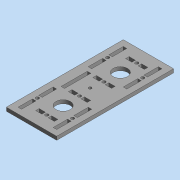
# Autodesk Inventor part: X-Anchor-Side
Saved by Autodesk Inventor 2016 SP1 (Build 200210100, 210)
## iProperties
Created: 2016-01-21
Part Number: X-Anchor-Side
Material: Generic
Document SubType Name: Modeling
Designer: Mohamed A.
Density: 1 g/cm^3
Appearance: Default
Author: Mohamed A.
Autodesk Inventor part; units mm, degrees
ref_plane "YZ Plane" through (0, 0, 0) normal (1, 0, 0) x (0, 1, 0)
ref_plane "XZ Plane" through (0, 0, 0) normal (0, 1, 0) x (-1, 0, 0)
ref_plane "XY Plane" through (0, 0, 0) normal (0, 0, 1) x (1, 0, 0)
sketch "Sketch1" plane through (0, 0, 0) normal (0, 0, 1) x (1, 0, 0)
  line L0 (21.5007, 49.9294) -> (-21.5007, 49.9294)
  line L1 (-21.5007, 49.9294) -> (-21.5007, -49.9294)
  line L2 (-21.5007, -49.9294) -> (21.5007, -49.9294)
  line L3 (21.5007, -49.9294) -> (21.5007, 49.9294)
  line L4 (-13.5007, 14.9765) -> (-16.5007, 14.9765)
  line L5 (-16.5007, 14.9765) -> (-16.5007, 27.3029)
  line L6 (-16.5007, 27.3029) -> (-13.5007, 27.3029)
  line L7 (-13.5007, 27.3029) -> (-13.5007, 14.9765)
  line L8 (-13.5007, -27.3029) -> (-16.5007, -27.3029)
  line L9 (-16.5007, -27.3029) -> (-16.5007, -14.9765)
  line L10 (-16.5007, -14.9765) -> (-13.5007, -14.9765)
  line L11 (-13.5007, -14.9765) -> (-13.5007, -27.3029)
  line L12 (-13.5007, -44.9294) -> (-16.5007, -44.9294)
  line L13 (-16.5007, -44.9294) -> (-16.5007, -32.6029)
  line L14 (-16.5007, -32.6029) -> (-13.5007, -32.6029)
  line L15 (-13.5007, -32.6029) -> (-13.5007, -44.9294)
  line L16 (-16.5007, 44.9294) -> (-13.5007, 44.9294)
  line L17 (-13.5007, 44.9294) -> (-13.5007, 32.6029)
  line L18 (-13.5007, 32.6029) -> (-16.5007, 32.6029)
  line L19 (-16.5007, 32.6029) -> (-16.5007, 44.9294)
  line L20 (-10.5007, -11.2324) -> (-13.5007, -11.2324)
  line L21 (-13.5007, -11.2324) -> (-13.5007, 11.2324)
  line L22 (-13.5007, 11.2324) -> (-10.5007, 11.2324)
  line L23 (-10.5007, 11.2324) -> (-10.5007, -11.2324)
  line L24 (16.5007, 14.9765) -> (13.5007, 14.9765)
  line L25 (13.5007, 14.9765) -> (13.5007, 27.3029)
  line L26 (13.5007, 27.3029) -> (16.5007, 27.3029)
  line L27 (16.5007, 27.3029) -> (16.5007, 14.9765)
  line L28 (16.5007, -27.3029) -> (13.5007, -27.3029)
  line L29 (13.5007, -27.3029) -> (13.5007, -14.9765)
  line L30 (13.5007, -14.9765) -> (16.5007, -14.9765)
  line L31 (16.5007, -14.9765) -> (16.5007, -27.3029)
  line L32 (16.5007, -44.9294) -> (13.5007, -44.9294)
  line L33 (13.5007, -44.9294) -> (13.5007, -32.6029)
  line L34 (13.5007, -32.6029) -> (16.5007, -32.6029)
  line L35 (16.5007, -32.6029) -> (16.5007, -44.9294)
  line L36 (13.5007, 44.9294) -> (16.5007, 44.9294)
  line L37 (16.5007, 44.9294) -> (16.5007, 32.6029)
  line L38 (16.5007, 32.6029) -> (13.5007, 32.6029)
  line L39 (13.5007, 32.6029) -> (13.5007, 44.9294)
  line L40 (4.1498, 36.9294) -> (4.1498, 39.9294)
  line L41 (4.1498, 39.9294) -> (9.5001, 39.9294)
  line L42 (9.5001, 39.9294) -> (9.5001, 36.9294)
  line L43 (9.5001, 36.9294) -> (4.1498, 36.9294)
  line L44 (-6.5006, 36.9294) -> (-6.5006, 39.9294)
  line L45 (-6.5006, 39.9294) -> (-1.1502, 39.9294)
  line L46 (-1.1502, 39.9294) -> (-1.1502, 36.9294)
  line L47 (-1.1502, 36.9294) -> (-6.5006, 36.9294)
  line L48 (-1.1502, 11.9294) -> (-1.1502, 8.9294)
  line L49 (-1.1502, 8.9294) -> (-6.5006, 8.9294)
  line L50 (-6.5006, 8.9294) -> (-6.5006, 11.9294)
  line L51 (-6.5006, 11.9294) -> (-1.1502, 11.9294)
  line L52 (9.5001, 11.9294) -> (9.5001, 8.9294)
  line L53 (9.5001, 8.9294) -> (4.1498, 8.9294)
  line L54 (4.1498, 8.9294) -> (4.1498, 11.9294)
  line L55 (4.1498, 11.9294) -> (9.5001, 11.9294)
  line L56 (4.1498, -11.9294) -> (4.1498, -8.9294)
  line L57 (4.1498, -8.9294) -> (9.5001, -8.9294)
  line L58 (9.5001, -8.9294) -> (9.5001, -11.9294)
  line L59 (9.5001, -11.9294) -> (4.1498, -11.9294)
  line L60 (-6.5006, -11.9294) -> (-6.5006, -8.9294)
  line L61 (-6.5006, -8.9294) -> (-1.1502, -8.9294)
  line L62 (-1.1502, -8.9294) -> (-1.1502, -11.9294)
  line L63 (-1.1502, -11.9294) -> (-6.5006, -11.9294)
  line L64 (4.1498, -39.9294) -> (4.1498, -36.9294)
  line L65 (4.1498, -36.9294) -> (9.5001, -36.9294)
  line L66 (9.5001, -36.9294) -> (9.5001, -39.9294)
  line L67 (9.5001, -39.9294) -> (4.1498, -39.9294)
  line L68 (-6.5006, -39.9294) -> (-6.5006, -36.9294)
  line L69 (-6.5006, -36.9294) -> (-1.1502, -36.9294)
  line L70 (-1.1502, -36.9294) -> (-1.1502, -39.9294)
  line L71 (-1.1502, -39.9294) -> (-6.5006, -39.9294)
  circle A0 centre (1.4998, 38.4294) radius 1.4
  line L72 (1.4998, 41.6656) -> (1.4998, 35.5125) construction
  circle A1 centre (1.4998, 10.4294) radius 1.4
  circle A2 centre (1.4998, -10.4294) radius 1.4
  circle A3 centre (1.4998, -38.4294) radius 1.4
  line L73 (-16.5007, 29.9529) -> (-13.5007, 29.9529) construction
  circle A4 centre (-15.0007, 29.9529) radius 1.4
  circle A5 centre (15.0007, 29.9529) radius 1.4
  line L74 (-16.5007, -29.9529) -> (-13.6007, -29.9529) construction
  circle A6 centre (-15.0507, -29.9529) radius 1.4
  circle A7 centre (15.0007, -29.9529) radius 1.4
  circle A8 centre (1.5007, -24.4294) radius 6.096
  circle A9 centre (1.5007, 24.4294) radius 6.096
  circle A10 centre (0, 0) radius 1.25
  dimension "d5" = 99.8588
  dimension "d6" = 43.0015
  dimension "d7" = 2.8
  dimension "d8" = 5.3
  dimension "d9" = 2.65
  dimension "d10" = 2.8
  dimension "d11" = 2.8
  dimension "d12" = 2.8
  dimension "d13" = 2.8
  dimension "d14" = 2.8
  dimension "d15" = 5.3
  dimension "d16" = 2.65
  dimension "d17" = 5.3
  dimension "d18" = 2.65
  dimension "d19" = 2.8
  dimension "d20" = 2.8
  dimension "d22" = 2.5
  constraints: 150 end point, 38 horizontal, 37 vertical, 11 centre point, 2 midpoint, 2 parallel, 1 coincident, 1 perpendicular, 1 point on line, 75 other
  measures "d5" distance between parallel lines of L2 L0
  measures "d6" distance between parallel lines of L3 L1
  measures "d7" diameter of A0
  measures "d8" distance between parallel lines of L40 L46
  measures "d9" distance between parallel lines of L72 L46
  measures "d10" diameter of A1
  measures "d11" diameter of A2
  measures "d12" diameter of A3
  measures "d13" diameter of A4
  measures "d14" diameter of A5
  measures "d15" distance between parallel lines of L6 L18
  measures "d16" distance between parallel lines of L6 L73
  measures "d17" distance between parallel lines of L14 L8
  measures "d18" distance between parallel lines of L14 L74
  measures "d19" diameter of A6
  measures "d20" diameter of A7
  measures "d22" diameter of A10
extrude "Extrusion1" add sketch "Sketch1" along normal blind 3
equation "\"d9\" = 0.5 * d8"
equation "\"d16\" = 0.5 * d15"
equation "\"d18\" = 0.5 * d17"
body "Solid1"
